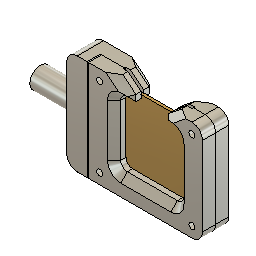
Elara 4th axis 2mm jig v3 (Autodesk Fusion 360 design; units mm, degrees)
Autodesk Fusion 360 part; units mm, degrees
note: some values were not read from the file. Set by a fixed rule: which sketch regions a step uses.
sketch "Sketch1" plane through (0, 0, 0) normal (0, 0, 1) x (1, 0, 0)
  line L0 (8, 0) -> (95, 0)
  line L1 (103, 8) -> (103, 68.2)
  line L2 (95, 76.2) -> (8, 76.2)
  line L3 (0, 68.2) -> (0, 8)
  circle A0 centre (60, 38.1) radius 23.3625 construction
  circle A1 centre (60, 38.1) radius 18.6 construction
  circle A2 centre (60, 38.1) radius 24
  line L4 (34.6, 63.5) -> (85.4, 63.5) construction
  line L5 (85.4, 63.5) -> (85.4, 12.7) construction
  line L6 (85.4, 12.7) -> (34.6, 12.7) construction
  line L7 (34.6, 12.7) -> (34.6, 63.5) construction
  arc A3 (103, 68.2) -> (95, 76.2) centre (95, 68.2) ccw
  arc A4 (95, 0) -> (103, 8) centre (95, 8) ccw
  circle A5 centre (95, 68.2) radius 1.65
  circle A6 centre (95, 8) radius 1.65
  circle A7 centre (25, 68.2) radius 1.65
  circle A8 centre (25, 8) radius 1.65
  line L8 (0, 38.1) -> (-50, 38.1) construction
  line L9 (47.5, 58.5878) -> (47.5, 76.2)
  line L10 (72.5, 58.5878) -> (72.5, 76.2)
  line L11 (60, 38.1) -> (60, 76.2) construction
  line L12 (16, 76.2) -> (16, 0)
  line L13 (0, 46.1) -> (-30, 46.1)
  line L14 (-30, 46.1) -> (-30, 38.1)
  line L15 (-30, 38.1) -> (0, 38.1)
  line L16 (33.8, 0) -> (33.8, 76.2)
  line L17 (86.2, 0) -> (86.2, 76.2)
  line L18 (15.5, 0) -> (15.5, 76.2)
  line L19 (16.5, 0) -> (16.5, 76.2)
  circle A9 centre (25, 68.2) radius 2.25
  circle A10 centre (95, 68.2) radius 2.25
  circle A11 centre (95, 8) radius 2.25
  circle A12 centre (25, 8) radius 2.25
  line L20 (47.5, 68.2) -> (37.5, 76.2)
  line L21 (72.5, 68.2) -> (82.5, 76.2)
  line L22 (34.6, 76.2) -> (34.6, 0)
  line L23 (85.4, 0) -> (85.4, 76.2)
  line L24 (33.8, 10.1) -> (86.2, 10.1)
  line L25 (33.8, 66.1) -> (86.2, 66.1)
  arc A13 (33.8, 10.1) -> (43.8, 10.1) centre (38.8, 10.1) ccw
  arc A14 (76.2, 10.1) -> (86.2, 10.1) centre (81.2, 10.1) ccw
  arc A15 (8, 76.2) -> (0, 68.2) centre (8, 68.2) ccw
  arc A16 (0, 8) -> (8, 0) centre (8, 8) ccw
  line L26 (103.9728, 65.6083) -> (118.9039, 65.6806) construction
  line L27 (118.9039, 65.6806) -> (118.8893, 68.6863) construction
  line L28 (118.8893, 68.6863) -> (103.9583, 68.614) construction
  line L29 (103.9583, 68.614) -> (103.9728, 65.6083) construction
  line L30 (0.7334, -6.4335) -> (20.3258, -6.3506) construction
  line L31 (20.3258, -6.3506) -> (20.3131, -3.3448) construction
  line L32 (20.3131, -3.3448) -> (0.7207, -3.4278) construction
  line L33 (0.7207, -3.4278) -> (0.7334, -6.4335) construction
  line L34 (-18.6738, 11.9015) -> (0.9186, 11.9844) construction
  line L35 (0.9186, 11.9844) -> (0.9059, 14.9901) construction
  line L36 (0.9059, 14.9901) -> (-18.6865, 14.9072) construction
  line L37 (-18.6865, 14.9072) -> (-18.6738, 11.9015) construction
  line L38 (-9.6516, 2.3848) -> (13.035, 2.4962) construction
  line L39 (13.035, 2.4962) -> (13.0067, 8.2636) construction
  line L40 (13.0067, 8.2636) -> (-9.6799, 8.1522) construction
  line L41 (-9.6799, 8.1522) -> (-9.6516, 2.3848) construction
  line L42 (0, 38.1) -> (28, 38.1) construction
  line L43 (41, 63.5) -> (79, 63.5)
  line L44 (84, 58.5) -> (84, 19.1)
  line L45 (79, 14.1) -> (41, 14.1)
  line L46 (36, 19.1) -> (36, 58.5)
  arc A17 (41, 63.5) -> (36, 58.5) centre (41, 58.5) ccw
  arc A18 (84, 58.5) -> (79, 63.5) centre (79, 58.5) ccw
  arc A19 (79, 14.1) -> (84, 19.1) centre (79, 19.1) ccw
  arc A20 (36, 19.1) -> (41, 14.1) centre (41, 19.1) ccw
  point P0 (0, 76.2)
  point P1 (34.6, 38.1)
  point P2 (60, 63.5)
  point P3 (84, 14.1)
  point P4 (36, 14.1)
  dimension "d1" = 37.2
  dimension "d3" = 4.7625
  dimension "d4" = 48
  dimension "d5" = 76.2
  dimension "d6" = 38.1
  dimension "d7" = 43
  dimension "d8" = 60
  dimension "d9" = 50.8
  dimension "d10" = 50.8
  dimension "d11" = 8
  dimension "d12" = 8
  dimension "d13" = 3.3
  dimension "d14" = 3.3
  dimension "d15" = 3.3
  dimension "d16" = 3.3
  dimension "d17" = 35
  dimension "d18" = 35
  dimension "d19" = 50
  dimension "d20" = 12.5
  dimension "d21" = 12.5
  dimension "d22" = 12.7
  dimension "d25" = 9
  dimension "d29" = 8
  dimension "d31" = 30
  dimension "d35" = 26.2
  dimension "d36" = 26.2
  dimension "d44" = 0.5
  dimension "d45" = 0.5
  dimension "d46" = 4.5
  dimension "d47" = 4.5
  dimension "d48" = 4.5
  dimension "d49" = 4.5
  dimension "d50" = 8
  dimension "d51" = 10
  dimension "d55" = 10
  dimension "d56" = 8
  dimension "d57" = 25.4
  dimension "d58" = 25.4
  dimension "d65" = 28
  dimension "d66" = 28
  dimension "d67" = 5
  dimension "d68" = 5
  dimension "d69" = 8
  dimension "d70" = 8
  dimension "d71" = 2
  dimension "d73" = 2
  dimension "d74" = 2
  dimension "d76" = 2
  dimension "d77" = 24
  dimension "d78" = 48
  dimension "d79" = 24
  dimension "d80" = 5
  constraint horizontal L0
  constraint vertical L1
  constraint horizontal L2
  constraint vertical L3
  constraint concentric A0 A1
  constraint concentric A1 A2
  constraint horizontal L4
  constraint vertical L5
  constraint horizontal L6
  constraint vertical L7
  constraint tangent L1 A3
  constraint tangent L2 A3
  constraint tangent L0 A4
  constraint tangent L1 A4
  constraint concentric A3 A5
  constraint concentric A4 A6
  constraint horizontal A3.centre A7.centre
  constraint horizontal A4.centre A8.centre
  constraint vertical A7.centre A8.centre
  constraint perpendicular L3 L8
  constraint midpoint L7 P1
  constraint midpoint L4 P2
  constraint vertical A0.centre P2
  constraint horizontal A0.centre P1
  constraint coincident A2 L9.start
  constraint coincident L2 L9.end
  constraint perpendicular L2 L9
  constraint coincident A2 L10.start
  constraint coincident L2 L10.end
  constraint perpendicular L2 L10
  constraint coincident A0.centre A1.centre
  constraint coincident L2 L11.end
  constraint perpendicular L2 L11
  constraint coincident L2 L12.start
  constraint coincident L0 L12.end
  constraint perpendicular L0 L12
  constraint coincident L3 L13.start
  constraint perpendicular L3 L13
  constraint coincident L8 L14.end
  constraint perpendicular L8 L14
  constraint coincident L0 L16.start
  constraint coincident L2 L16.end
  constraint perpendicular L2 L16
  constraint coincident L0 L17.start
  constraint coincident L2 L17.end
  constraint perpendicular L2 L17
  constraint coincident L0 L18.start
  constraint coincident L2 L18.end
  constraint perpendicular L2 L18
  constraint coincident L0 L19.start
  constraint coincident L2 L19.end
  constraint perpendicular L2 L19
  constraint concentric A7 A9
  constraint concentric A5 A10
  constraint concentric A6 A11
  constraint concentric A8 A12
  constraint coincident L9 L20.start
  constraint coincident L2 L20.end
  constraint coincident L10 L21.start
  constraint coincident L2 L21.end
  constraint coincident L2 L22.start
  constraint coincident L0 L22.end
  constraint perpendicular L0 L22
  constraint coincident L0 L23.start
  constraint coincident L2 L23.end
  constraint perpendicular L2 L23
  constraint coincident L16 L24.start
  constraint coincident L17 L24.end
  constraint perpendicular L17 L24
  constraint coincident L16 L25.start
  constraint coincident L17 L25.end
  constraint perpendicular L17 L25
  constraint tangent L16 A13
  constraint coincident L24 A13.end
  constraint tangent L17 A14
  constraint coincident L24 A14.start
  constraint coincident L3 L8.start
  constraint coincident P0 L2
  constraint coincident P0 L3
  constraint tangent L2 A15
  constraint tangent L3 A15
  constraint coincident origin L0
  constraint coincident origin L3
  constraint tangent L0 A16
  constraint tangent L3 A16
  constraint perpendicular L19 L42
  constraint horizontal L43
  constraint vertical L44
  constraint horizontal L45
  constraint vertical L46
  constraint tangent L43 A17
  constraint tangent L46 A17
  constraint tangent L43 A18
  constraint tangent L44 A18
  constraint equal A17 A18
  constraint coincident P3 L44
  constraint coincident P3 L45
  constraint tangent L44 A19
  constraint tangent L45 A19
  constraint equal A17 A19
  constraint coincident P4 L45
  constraint coincident P4 L46
  constraint tangent L45 A20
  constraint tangent L46 A20
  constraint equal A17 A20
  measures "d1" diameter of A1
  measures "d3" distance of A0 A1
  measures "d4" diameter of A2
  measures "d5" distance of origin P0
  measures "d6" distance of L0 A0.centre
  measures "d7" distance of L1 A0.centre
  measures "d8" distance of L3 A0.centre
  measures "d9" distance of L4.end L5.end
  measures "d10" distance of L4.start L4.end
  measures "d11" radius of A3
  measures "d12" radius of A4
  measures "d13" diameter of A6
  measures "d14" diameter of A5
  measures "d15" diameter of A7
  measures "d16" diameter of A8
  measures "d17" horizontal distance of A0.centre A4.centre
  measures "d18" horizontal distance of A0.centre A8.centre
  measures "d19" distance of L8.start L8.end
  measures "d20" distance of L9 L11
  measures "d21" distance of L10 L11
  measures "d22" distance of L2 L4
  measures "d25" distance of A8.centre L12
  measures "d29" distance of L8 L13
  measures "d31" distance of L13.start L13.end
  measures "d35" distance of L11 L16
  measures "d36" distance of L11 L17
  measures "d44" distance of L12 L19
  measures "d45" distance of L12 L18
  measures "d46" diameter of A12
  measures "d47" diameter of A11
  measures "d48" diameter of A10
  measures "d49" diameter of A9
  measures "d50" distance of L9.end L20.start
  measures "d51" distance of L9.end L20.end
  measures "d55" distance of L10.end L21.end
  measures "d56" distance of L10.end L21.start
  measures "d57" distance of L11 L22
  measures "d58" distance of L11 L23
  measures "d65" distance of A0.centre L24
  measures "d66" distance of A0.centre L25
  measures "d67" radius of A13
  measures "d68" radius of A14
  measures "d69" radius of A15
  measures "d70" radius of A16
  measures "d77" distance of L11 L44
  measures "d78" distance of P3 P4
  measures "d79" distance of P1 L45
  measures "d80" radius of A17
extrude "Extrude1" add sketch "Sketch1" against normal blind 10 contours L0 L2 L3 L18 A15 A16 | L0 L2 L12 L18 | L0 L2 L12 L19 | L0 L2 L16 L19 | L0 L16 L22 A13 | L0 L22 L23 L24 A13 A14 | L16 L22 L24 L25 | L22 L24 A13 | L2 L16 L22 L25 | L0 L17 L23 A14 | L22 L24 A13 | L9 L10 L22 L23 L24 L25 L43 L44 L45 L46 A17 A18 A19 A20 | L2 L9 L20 L22 L25 | L0 L1 L2 A3 A4 L17 | L23 L24 A14 | L23 L24 A14 | L17 L23 L24 L25 | L2 L17 L23 L25 | L2 L10 L21 L23 L25 | A9 | A10 | A11 | A12 makes body 1
extrude "Extrude2" add sketch "Sketch1" along normal blind 10 contours L0 L2 L3 L18 A15 A16 bodies 1
revolve "Revolve1" add sketch "Sketch1" angle 360 about axis through (0, 38.1, 0) along (-1, 0, 0) contours L3 L13 L14 L15 bodies 1
extrude "Extrude3" cut sketch "Sketch1" against normal blind 1.02 contours L16 L22 L24 L25 | L22 L24 A13 | L2 L16 L22 L25 | L22 L24 A13 | L9 L10 L22 L23 L24 L25 L43 L44 L45 L46 A17 A18 A19 A20 | L2 L9 L20 L22 L25 | L23 L24 A14 | L23 L24 A14 | L2 L9 L20 | L17 L23 L24 L25 | L2 L17 L23 L25 | L2 L10 L21 L23 L25 | A2 L9 L43 L46 A17 | L2 L10 L21 | A2 L10 L43 L44 A18 | A2 L45 L46 A20 | A2 L44 L45 A19 bodies 1
extrude "Extrude4" add sketch "Sketch1" along normal blind 10 separate body contours L0 L2 L16 L19 | L0 L16 L22 A13 | L0 L22 L23 L24 A13 A14 | L16 L22 L24 L25 | L22 L24 A13 | L2 L16 L22 L25 | L0 L17 L23 A14 | L22 L24 A13 | L9 L10 L22 L23 L24 L25 L43 L44 L45 L46 A17 A18 A19 A20 | L2 L9 L20 L22 L25 | L0 L1 L2 A3 A4 L17 | L23 L24 A14 | L23 L24 A14 | L17 L23 L24 L25 | L2 L17 L23 L25 | L2 L10 L21 L23 L25 makes body 2
extrude "Extrude5" cut sketch "Sketch1" along normal blind 1.02 contours L16 L22 L24 L25 | L22 L24 A13 | L2 L16 L22 L25 | L22 L24 A13 | L9 L10 L22 L23 L24 L25 L43 L44 L45 L46 A17 A18 A19 A20 | L2 L9 L20 L22 L25 | L23 L24 A14 | L23 L24 A14 | L2 L9 L20 | L17 L23 L24 L25 | L2 L17 L23 L25 | L2 L10 L21 L23 L25 | A2 L9 L43 L46 A17 | L2 L10 L21 | A2 L10 L43 L44 A18 | A2 L45 L46 A20 | A2 L44 L45 A19 bodies 2
chamfer "Chamfer1" distance 5 angle 45 26 edges at (42.5, 72.2, 10) (47.5, 65.85, 10) (44.25, 63.5, 10) (75.75, 63.5, 10) (82.5355, 62.0355, 10) (84, 38.8, 10) (82.5355, 15.5645, 10) (60, 14.1, 10) (37.4645, 15.5645, 10) (36, 38.8, 10) (37.4645, 62.0355, 10) (72.5, 65.85, 10) (77.5, 72.2, 10) (42.5, 72.2, -10) (47.5, 65.85, -10) (37.4645, 62.0355, -10) (36, 38.8, -10) (37.4645, 15.5645, -10) (60, 14.1, -10) (82.5355, 15.5645, -10) (84, 38.8, -10) (82.5355, 62.0355, -10) (75.75, 63.5, -10) (44.25, 63.5, -10) (72.5, 65.85, -10) (77.5, 72.2, -10) on bodies 1 2
extrude "Extrude6" add sketch "Sketch1" along normal blind 1.05 and the other way blind 1.05 separate body contours L9 L10 L22 L23 L24 L25 L43 L44 L45 L46 A17 A18 A19 A20 | L9 L10 L25 L43 | A2 L9 L10 L43 | A2 L9 L43 L46 A17 | A2 | A2 L10 L43 L44 A18 | A2 L45 L46 A20 | A2 L44 L45 A19 makes body 3
equation "d3 = 0.125 in + 0.0625 in"
equation "d6 = ( 76.2 / 2 ) * 1 mm"
